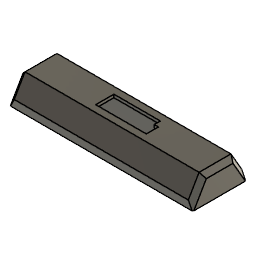
Smart Fan Shroud Top (Autodesk Fusion 360 design; units mm, degrees)
part number: 2026-06-19-13-26-21-851
Autodesk Fusion 360 part; units mm, degrees
sketch "Sketch1" plane through (0, 0, 0) normal (0, 0, 1) x (1, 0, 0)
  line L0 (0, 0) -> (120, 0)
  line L1 (120, 0) -> (120, 35)
  line L2 (120, 35) -> (0, 35)
  line L3 (0, 35) -> (0, 0)
  dimension "d1" = 120
  dimension "d2" = 35
  constraint horizontal L0
  constraint vertical L1
  constraint horizontal L2
  constraint vertical L3
  constraint coincident L0.start L3.end
  measures "d1" distance of L0.start L0.end
  measures "d2" distance of L0.start L2.end
extrude "Extrude1" add sketch "Sketch1" along normal blind 17.2
chamfer "Chamfer1" distance 7.0437 angle 60 2 edges at (60, 0, 17.2) (60, 35, 17.2) measured on face at (40, 23.3333, 17.2) measured on face at (40, 23.3333, 17.2)
chamfer "Chamfer2" distance 3 angle 45 6 edges at (0, 3.5218, 11.1) (0, 31.4782, 11.1) (0, 17.5, 17.2) (120, 17.5, 17.2) (120, 3.5218, 11.1) (120, 31.4782, 11.1) measured on face at (40, 4.6958, 13.1333) measured on face at (80, 30.3042, 13.1333) measured on face at (40, 20.9854, 17.2) measured on face at (40, 20.9854, 17.2) measured on face at (40, 4.6958, 13.1333) measured on face at (80, 30.3042, 13.1333)
sketch "Sketch2" plane through (0, 0, 0) normal (0, 0, -1) x (1, 0, 0)
  line L0 (0, -0.5773) -> (0, -34.4227)
  line L1 (120, -34.4227) -> (120, -0.5773)
  line L2 (115.1, -7.4) -> (4.9, -7.4)
  line L3 (4.9, -7.4) -> (4.9, -27.6)
  line L4 (4.9, -27.6) -> (115.1, -27.6)
  line L5 (115.1, -27.6) -> (115.1, -7.4)
  line L6 (115.1, -7.4) -> (4.9, -27.6) construction
  line L7 (4.9, -7.4) -> (115.1, -27.6) construction
  line L8 (120, -0.5773) -> (119.5, 0)
  line L9 (0.5, 0) -> (0, -0.5773)
  line L10 (0, -34.4227) -> (0.5, -35)
  line L11 (119.5, -35) -> (120, -34.4227)
  line L12 (60, 0) -> (60, -35) construction
  line L13 (119.5, 0) -> (0.5, 0)
  line L14 (0.5, -35) -> (119.5, -35)
  point P0 (60, -17.5)
  dimension "d9" = 110.2
  dimension "d10" = 20.2
  constraint horizontal L2
  constraint perpendicular L2 L3
  constraint parallel L2 L4
  constraint parallel L3 L5
  constraint coincident L6 P0
  constraint coincident L7 P0
  constraint midpoint P0 L12
  measures "d9" distance of L3.end L4.end
  measures "d10" distance of L2.end L3.end
extrude "Extrude2" cut sketch "Sketch2" against normal blind 15.2 contours L2 L3 L4 L5
sketch "Sketch3" plane through (0, 0, 17.2) normal (0, 0, 1) x (-1, 0, 0)
  line L0 (-117, -7.0437) -> (-117, -27.9563)
  line L1 (-117, -27.9563) -> (-3, -27.9563)
  line L2 (-3, -27.9563) -> (-3, -7.0437)
  line L3 (-3, -7.0437) -> (-117, -7.0437)
  line L4 (-60, -27.9563) -> (-60, -7.0437) construction
  line L5 (-117, -17.5) -> (-3, -17.5) construction
  line L6 (-44.8, -11.55) -> (-75.2, -11.55)
  line L7 (-75.2, -11.55) -> (-75.2, -23.45)
  line L8 (-75.2, -23.45) -> (-44.8, -23.45)
  line L9 (-44.8, -23.45) -> (-44.8, -11.55)
  line L10 (-75.2, -11.55) -> (-77.95, -11.55)
  line L11 (-77.95, -11.55) -> (-77.95, -19.45)
  line L12 (-77.95, -19.45) -> (-75.2, -19.45)
  line L13 (-75.2, -19.45) -> (-75.2, -11.55)
  line L14 (-60, -23.45) -> (-60, -11.55) construction
  dimension "d13" = 30.4
  dimension "d14" = 11.9
  dimension "d15" = 2.75
  dimension "d16" = 7.9
  constraint midpoint L1 L4.start
  constraint midpoint L3 L4.end
  constraint midpoint L0 L5.start
  constraint midpoint L2 L5.end
  constraint horizontal L6
  constraint vertical L7
  constraint horizontal L8
  constraint vertical L9
  constraint horizontal L10
  constraint vertical L11
  constraint horizontal L12
  constraint vertical L13
  constraint midpoint L8 L14.start
  constraint midpoint L6 L14.end
  constraint midpoint L4 L14
  measures "d13" distance of L6.start L6.end
  measures "d14" distance of L6.start L8.end
  measures "d15" distance of L6.end L10.end
  measures "d16" distance of L6.end L12.end
extrude "Extrude3" cut sketch "Sketch3" against normal blind 2 contours L6 L7 L8 L9 L13 | L7 L10 L11 L12 L13
equation "d3 = 10 mm - 2.8 mm + 5 mm + 5 mm"
equation "d11 = -5.2 mm - 5 mm - 5 mm"
equation "d13 = 30 mm + 0.4 mm"
equation "d14 = 11.5 mm + 0.4 mm"
equation "d16 = 7.5 mm + 0.4 mm"
